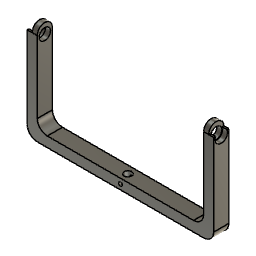
Pos29 (Autodesk Fusion 360 design; units mm, degrees)
Autodesk Fusion 360 part; units mm, degrees
note: some values were not read from the file. Set by a fixed rule: the direction of a hole.
sketch "Sketch1" plane through (0, 0, 0) normal (0, 1, 0) x (1, 0, 0)
  line L0 (0, 0) -> (66, 0)
  line L1 (0, 0) -> (0, -8) construction
  line L2 (74, -8) -> (74, -73)
  line L3 (74, -73) -> (70, -73)
  line L4 (70, -73) -> (70, -79)
  line L5 (70, -79) -> (66, -79)
  line L6 (66, -79) -> (66, -16)
  line L7 (58, -8) -> (0, -8)
  arc A0 (66, -16) -> (58, -8) centre (58, -16) ccw
  arc A1 (74, -8) -> (66, 0) centre (66, -8) ccw
  line L8 (-58, -8) -> (0, -8)
  line L9 (0, 0) -> (-66, 0)
  arc A2 (-66, 0) -> (-74, -8) centre (-66, -8) ccw
  line L10 (-74, -8) -> (-74, -73)
  arc A3 (-58, -8) -> (-66, -16) centre (-58, -16) ccw
  line L11 (-66, -79) -> (-66, -16)
  line L12 (-70, -79) -> (-66, -79)
  line L13 (-70, -73) -> (-70, -79)
  line L14 (-74, -73) -> (-70, -73)
  circle A4 centre (0, -4) radius 1.5
  point P0 (74, 0)
  point P1 (66, -8)
  dimension "d1" = 74
  dimension "d2" = 8
  dimension "d3" = 73
  dimension "d4" = 4
  dimension "d5" = 6
  dimension "d6" = 4
  dimension "d7" = 71
  dimension "d8" = 8
  dimension "d9" = 8
  dimension "d10" = 3
  constraint coincident L0.start L1.start
  constraint horizontal L0
  constraint perpendicular L0 L1
  constraint perpendicular L0 L2
  constraint perpendicular L2 L3
  constraint perpendicular L3 L4
  constraint perpendicular L4 L5
  constraint perpendicular L5 L6
  constraint coincident P1 L6
  constraint coincident P1 L7
  constraint tangent L6 A0
  constraint tangent L7 A0
  constraint coincident P0 L0
  constraint coincident P0 L2
  constraint tangent L0 A1
  constraint tangent L2 A1
  constraint symmetric L0.start L1 L9.start
  constraint symmetric L7.end L1 L8.end
  constraint symmetric L1 L2.end L10.end
  constraint symmetric L1 L3.end L13.start
  constraint symmetric L1 L4.end L12.start
  constraint symmetric L1 L5.end L11.start
  constraint symmetric L1 L6.end A3.end
  constraint symmetric L1 L7.start L8.start
  constraint symmetric L1 A0 A3
  constraint symmetric L1 L0.end L9.end
  constraint symmetric L1 L2.start A2.end
  constraint symmetric L1 A1 A2
  constraint midpoint L1 A4.centre
  measures "d1" distance of L0.start P0
  measures "d2" distance of L0.start L1.end
  measures "d3" distance of P0 L2.end
  measures "d4" distance of L2.end L3.end
  measures "d5" distance of L3.end L4.end
  measures "d6" distance of L4.end L5.end
  measures "d7" distance of L5.end P1
  measures "d8" radius of A0
  measures "d9" radius of A1
  measures "d10" diameter of A4
extrude "Extrude1" add sketch "Sketch1" along normal blind 12
fillet "Fillet1" radius 6 4 edges at (68, 12, 79) (68, 0, 79) (-68, 12, 79) (-68, 0, 79)
sketch "Sketch2" plane through (-74, 0, 0) normal (1, 0, 0) x (0, 1, 0)
  arc A0 (12, 73) -> (0, 73) centre (6, 73) ccw
  line L0 (0, 73) -> (0, 16)
  line L1 (0, 16) -> (12, 16)
  line L2 (12, 16) -> (12, 73)
  line L3 (6, 16) -> (6, 71) construction
  circle A1 centre (6, 71) radius 4.5
  line L4 (0, 8) -> (0, 73)
  line L5 (0, 73) -> (12, 73)
  line L6 (12, 73) -> (12, 8)
  line L7 (12, 8) -> (0, 8)
  dimension "d15" = 55
  dimension "d16" = 9
  constraint midpoint L1 L3.start
  constraint perpendicular L1 L3
  constraint coincident L3.end A1.centre
  measures "d15" distance of L3.start L3.end
  measures "d16" diameter of A1
hole "Hole1" at (-74, 6, 71) direction (1, 0, 0) diameter 9 depth 10 tip angle 118 counterbore diameter 10 counterbore depth 4
mirror "Mirror1" about plane through (0, 0, 0) normal (1, 0, 0) of "Hole1"
sketch "Sketch3" plane through (0, 0, 8) normal (0, 0, 1) x (-1, 0, 0)
  line L0 (58, 0) -> (-58, 0)
  line L1 (-58, 0) -> (-58, -12)
  line L2 (-58, -12) -> (58, -12)
  line L3 (58, -12) -> (58, 0)
  line L4 (0, 0) -> (0, -6) construction
  circle A0 centre (0, -6) radius 3
  dimension "d24" = 6
  dimension "d25" = 6
  constraint coincident L4.start origin
  constraint perpendicular L0 L4
  constraint coincident L4.end A0.centre
  measures "d24" diameter of A0
  measures "d25" distance of L0 L4.end
hole "Hole2" at (0, 6, 8) direction (0, 0, -1) diameter 6 depth 10 tip angle 118
